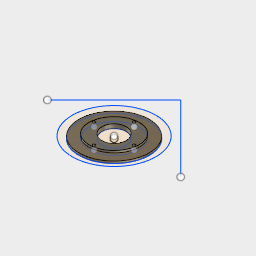
Emco PC Turn 55 Consew Motor Mount v12 (Autodesk Fusion 360 design; units mm, degrees)
Autodesk Fusion 360 part; units mm, degrees
sketch "Sketch12" plane through (0, 0, 0) normal (0, 0, 1) x (1, 0, 0)
  circle A0 centre (-29.9974, 0) radius 2
  circle A1 centre (29.9974, 0) radius 2
  circle A2 centre (0, -29.9974) radius 2
  ellipse E0 centre (0, 0) end of major axis (-25.1023, -25.1023) minor radius 31
  ellipse E1 centre (0, 0) end of major axis (-35.7089, -35.7089) minor radius 46
  circle A3 centre (0, 0) radius 18
  circle A4 centre (0, 29.9974) radius 2
  line L0 (-100, 0) -> (0, 100)
  line L1 (0, 100) -> (100, 0)
  point P0 (0, 29.9974)
  dimension "d4" = 0
  dimension "d5" = 0
  dimension "d6" = 0
  dimension "d7" = 0
  dimension "d28" = 36
  dimension "d33" = 35.5
  dimension "d34" = 31
  measures "d28" diameter of A3
  measures "d33" distance of E0
extrude "Extrude6" add sketch "Sketch12" along normal blind 6.35 contours E0
extrude "Extrude7" add sketch "Sketch12" along normal blind 3.175 contours E1
sketch "Sketch14" plane through (0, 0, 3.175) normal (0, 0, 1) x (-1, 0, 0)
  ellipse E0 centre (0, 0) end of major axis (25.1023, 25.1023) minor radius 31
  ellipse E1 centre (0, 0) end of major axis (35.7089, 35.7089) minor radius 46
  ellipse E2 centre (0, 0) end of major axis (42.78, 42.78) minor radius 56
